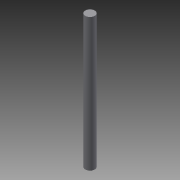
# Autodesk Inventor part: screw
Saved by Autodesk Inventor 2015 (Build 190159000, 159)
## iProperties
Created: 2015-01-12
Part Number: screw
Material: Generic
Document SubType Name: Modeling
Designer: whitaus15
Density: 1 g/cm^3
Appearance: Default
Author: whitaus15
Autodesk Inventor part; units mm, degrees
ref_plane "YZ Plane" through (0, 0, 0) normal (1, 0, 0) x (0, 1, 0)
ref_plane "XZ Plane" through (0, 0, 0) normal (0, 1, 0) x (-1, 0, 0)
ref_plane "XY Plane" through (0, 0, 0) normal (0, 0, 1) x (1, 0, 0)
sketch "Sketch1" plane through (0, 0, 0) normal (0, 1, 0) x (-1, 0, 0)
  circle A0 centre (0.0324, -0.0346) radius 0.9017
  point P0 (0, 0)
  dimension "d0" = 1.8034
  dimension "d0" = 1.8034
  constraints: 1 centre point
  measures "d0" diameter of A0
extrude "Extrusion1" add sketch "Sketch1" along normal blind 25.4
body "Solid1"
